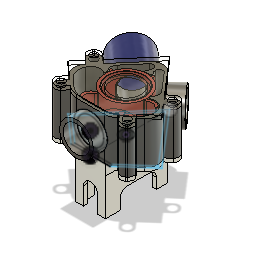
Air Transistor V4 (Autodesk Fusion 360 design; units mm, degrees)
Autodesk Fusion 360 part; units mm, degrees
sketch "Sketch1" plane through (0, 0, 0) normal (0, 1, 0) x (1, 0, 0)
  line L0 (-26.6187, 13.789) -> (0, 44.787)
  line L1 (-11, 0) -> (0, 0)
  line L2 (0, 44.787) -> (0, 0) construction
  line L3 (26.6187, 13.789) -> (0, 44.787)
  line L4 (11, 0) -> (0, 0)
  line L5 (-24.5168, 13.9343) -> (-10.4326, 1.5)
  line L6 (-26.6187, 13.789) -> (-11, 0)
  line L7 (-24.5168, 13.9343) -> (0, 42.4846)
  line L8 (-10.4326, 1.5) -> (0, 1.5)
  line L9 (24.5168, 13.9343) -> (10.4326, 1.5)
  line L10 (26.6187, 13.789) -> (11, 0)
  line L11 (10.4326, 1.5) -> (0, 1.5)
  line L12 (24.5168, 13.9343) -> (0, 42.4846)
  dimension "d70" = 1.5
  dimension "d71" = 1.5
  dimension "d72" = 22
  dimension "d73" = 1.5
  dimension "d85" = 0
  dimension "d86" = 0
  dimension "d87" = 0
  dimension "d88" = 0
  dimension "d121" = 0
  dimension "d122" = 0
  dimension "d123" = 0
  dimension "d124" = 0
  dimension "d131" = 0
  dimension "d132" = 0
  dimension "d133" = 0
  dimension "d134" = 0
  constraint coincident L1.end L2.end
  constraint horizontal L1
  constraint perpendicular L1 L2
  constraint symmetric L1.end L2 L4.end
  constraint symmetric L0.end L2 L3.end
  constraint parallel L5 L6
  constraint symmetric L2 L5.start L9.start
  constraint symmetric L2 L5.end L9.end
  constraint symmetric L2 L0.start L3.start
  constraint symmetric L2 L1.start L4.start
  constraint horizontal L8
  constraint horizontal L11
  constraint parallel L0 L7
  constraint parallel L3 L12
  measures "d70" distance of L5 L6
  measures "d71" distance of L0 L7
  measures "d72" distance of L1.start L4.start
  measures "d73" distance of L1 L8
extrude "Extrude1" add sketch "Sketch1" along normal blind 2 contours L5 L7 L8 L9 L11 L12 makes body 1
extrude "Extrude1'" add sketch "Sketch1" along normal blind 24 separate body makes body 2 in component "Casing"
ref_plane "WorkPlane1" through (0, 12, 0) normal (0, 0, 1) x (1, 0, 0)
sketch "Sketch2" plane through (0, 12, 0) normal (0, 0, 1) x (1, 0, 0)
  circle A0 centre (0, 0) radius 7.5
  circle A1 centre (0, 0) radius 9.5
  dimension "d9" = 15
  dimension "d10" = 2
  constraint coincident A0.centre A1.centre
  measures "d9" diameter of A0
  measures "d10" distance of A0 A1
extrude "Extrude3" add sketch "Sketch2" along normal blind 8 bodies 2 in component "Casing"
extrude "Extrude2" cut sketch "Sketch2" against normal blind 1.5 contours A0 bodies 2 in component "Casing"
ref_plane "WorkPlane2" through (13.3094, 12, -29.288) normal (0.758663, 0, -0.651483) x (-0.651483, 0, -0.758663)
sketch "Sketch3" plane through (13.3094, 12, -29.288) normal (0.758663, 0, -0.651483) x (-0.651483, 0, -0.758663)
  circle A0 centre (6.4293, 0) radius 7.5
  circle A1 centre (6.4293, 0) radius 9.5
  line L0 (0, 0) -> (60.3978, 0) construction
  line L1 (20.4293, -12) -> (20.4293, 12) construction
  dimension "d16" = 15
  dimension "d17" = 2
  dimension "d18" = 14
  constraint concentric A0 A1
  constraint coincident L0.start origin
  constraint horizontal L0
  constraint coincident A0.centre L0
  measures "d16" diameter of A0
  measures "d17" distance of A0 A1
  measures "d18" distance of A0.centre L1
extrude "Extrude4" add sketch "Sketch3" along normal blind 8 bodies 2 in component "Casing"
extrude "Extrude5" cut 1 faces at (7.7655, 9.2149, -35.7439) along direction (-0.758663, 0, 0.651483) blind 1.5 on bodies 2 bodies 2 in component "Casing"
ref_plane "WorkPlane3" through (-13.3094, 12, -29.288) normal (-0.758663, 0, -0.651483) x (-0.651483, 0, 0.758663)
sketch "Sketch4" plane through (-13.3094, 12, -29.288) normal (-0.758663, 0, -0.651483) x (-0.651483, 0, 0.758663)
  circle A0 centre (-6.4293, 0) radius 7.5
  circle A1 centre (-6.4293, 0) radius 9.5
  line L0 (0, 0) -> (-68.9221, 0) construction
  line L1 (-20.4293, -12) -> (-20.4293, 12) construction
  dimension "d24" = 15
  dimension "d25" = 2
  dimension "d26" = 14
  constraint concentric A0 A1
  constraint coincident L0.start origin
  constraint horizontal L0
  constraint coincident A0.centre L0
  measures "d24" diameter of A0
  measures "d25" distance of A0 A1
  measures "d26" distance of A0.centre L1
extrude "Extrude6" add sketch "Sketch4" along normal blind 8 bodies 2 in component "Casing"
extrude "Extrude7" cut 1 faces at (-8.723, 11.908, -34.6289) along direction (0.758663, 0, 0.651483) blind 1.5 on bodies 2 bodies 2 in component "Casing"
ref_plane "WorkPlane4" through (0, 2.5, -21.9923) normal (0, 1, 0) x (0, 0, 1)
sketch "Sketch5" plane through (0, 2.5, -33.891) normal (0, 1, 0) x (1, 0, 0)
  circle A0 centre (0, -13.7563) radius 12
  circle A1 centre (0, -13.7563) radius 10.5
  line L0 (0, 0) -> (0, -47.8942) construction
  dimension "d32" = 24
  dimension "d35" = 1.5
  constraint concentric A0 A1
  constraint coincident L0.start origin
  constraint vertical L0
  constraint coincident A0.centre L0
  measures "d32" diameter of A0
  measures "d35" distance of A0 A1
extrude "Extrude6'" add sketch "Sketch5" along normal blind 3 separate body contours A1 makes body 3
extrude "Extrude1''" add sketch "Sketch5" along normal up to surface (21.4 mm away) separate body makes body 4 in component "Exchanger"
ref_plane "WorkPlane6" through (0, 0, -21.9923) normal (0, 1, 0) x (1, 0, 0)
sketch "Sketch7" plane through (0, 0, -21.9857) normal (0, 1, 0) x (1, 0, 0)
  circle A0 centre (0, -1.8509) radius 3.5
  point P0 (0, -1.8509)
  dimension "d43" = 7
  constraint coincident P0 A0.centre
  measures "d43" diameter of A0
extrude "Extrude7'" cut sketch "Sketch7" along normal blind 2 bodies 1
copy_body "CutPasteBodies1" bodies 1 removing the originals makes body 5 in component "Casing"
copy_body "CutPasteBodies1'" bodies 3 removing the originals makes body 6 in component "Exchanger"
ref_plane "WorkPlane7" through (0, 5.5, -20.1347) normal (0, 1, 0) x (1, 0, 0)
sketch "Sketch8" plane through (0, 5.5, -20.1347) normal (0, 1, 0) x (1, 0, 0)
  circle A0 centre (0, 0) radius 3.5
  circle A1 centre (0, 0) radius 3.5
  constraint coincident A0.centre A1.centre
  constraint tangent A0 A1
extrude "Extrude2'" cut sketch "Sketch8" against normal blind 3 bodies 6 in component "Exchanger"
ref_plane "WorkPlane8" through (0, 21.1035, -30.6347) normal (0, 0, 1) x (-1, 0, 0)
sketch "Sketch9" plane through (0, 18.9317, -30.6347) normal (0, 0, 1) x (1, 0, 0)
  circle A0 centre (0, -5.7317) radius 8.5
  line L0 (0, 4.9683) -> (0, -16.4317) construction
  line L1 (-12, 4.9683) -> (12, 4.9683) construction
  line L2 (-8.5, -14.2317) -> (-6.5, -14.2317)
  line L3 (-6.5, -14.2317) -> (-6.5, 2.7683)
  line L4 (-6.5, 2.7683) -> (-8.5, 2.7683)
  line L5 (-8.5, 2.7683) -> (-8.5, -14.2317)
  line L6 (0, 2.7683) -> (-13.5085, 2.7683) construction
  line L7 (0, -14.2317) -> (-15.3531, -14.2317) construction
  line L8 (8.5, -14.2317) -> (6.5, -14.2317)
  line L9 (8.5, 2.7683) -> (8.5, -14.2317)
  line L10 (6.5, -14.2317) -> (6.5, 2.7683)
  line L11 (6.5, 2.7683) -> (8.5, 2.7683)
  point P0 (0, -16.4317)
  dimension "d56" = 17
  dimension "d232" = 2
  constraint coincident P0 L0.end
  constraint coincident L0.start L1
  constraint coincident L0 A0.centre
  constraint midpoint L0 A0.centre
  constraint coincident origin L0
  constraint horizontal L2
  constraint vertical L3
  constraint horizontal L4
  constraint vertical L5
  constraint tangent A0 L5
  constraint coincident L0 L6.start
  constraint coincident A0 L6.start
  constraint tangent A0 L6
  constraint coincident L0 L7.start
  constraint coincident A0 L7.start
  constraint tangent A0 L7
  constraint coincident L2.end L7
  constraint coincident L3.end L6
  constraint symmetric L0 L2.start L8.start
  constraint symmetric L0 L2.end L8.end
  constraint symmetric L0 L3.end L10.end
  constraint symmetric L0 L4.end L9.start
  measures "d56" diameter of A0
  measures "d232" distance of L3.end L4.end
extrude "Extrude3'" cut sketch "Sketch9" along normal mid plane 8 contours A0 L3 L10 bodies 4 in component "Exchanger"
ref_plane "WorkPlane10" through (0, 2, -21.9923) normal (0, 1, 0) x (0, 0, 1)
sketch "Sketch11" plane through (0, 2, -21.9857) normal (0, 1, 0) x (1, 0, 0)
  line L0 (-15.5611, 3.108) -> (-12.3, 0.1598)
  line L1 (-12.3, 0.1598) -> (-12.3, -1.8623)
  line L2 (-12.3, -1.8623) -> (-16.5628, 1.9915)
  line L3 (-16.5628, 1.9915) -> (-15.5611, 3.108)
  line L4 (0, 11.9053) -> (0, -35.9889)
  line L5 (12.3, 0.1598) -> (12.3, -1.8623)
  line L6 (15.5611, 3.108) -> (12.3, 0.1598)
  line L7 (12.3, -1.8623) -> (16.5628, 1.9915)
  line L8 (16.5628, 1.9915) -> (15.5611, 3.108)
  line L9 (-24.5168, -8.0514) -> (0, 20.4989)
  line L10 (-0.75, 19.6255) -> (-0.75, 11.9686)
  line L11 (-0.7497, 10.4669) -> (0, 10.5777)
  line L12 (0, 22.8013) -> (0, -21.9857)
  line L13 (0.75, 19.6255) -> (0.75, 11.9686)
  line L14 (0.7497, 10.4669) -> (0, 10.5777)
  line L15 (-0.75, 19.6255) -> (0, 20.4989)
  line L16 (0, 20.4989) -> (0.75, 19.6255)
  circle A0 centre (0, -1.8509) radius 12 construction
  line L17 (-0.7497, 10.4669) -> (-1.9495, 10.2897)
  line L18 (-1.9495, 10.2897) -> (-1.9495, 11.7897)
  line L19 (-1.9495, 11.7897) -> (-0.75, 11.9686)
  line L20 (1.9495, 11.7897) -> (0.75, 11.9686)
  line L21 (1.9495, 10.2897) -> (1.9495, 11.7897)
  line L22 (0.7497, 10.4669) -> (1.9495, 10.2897)
  line L23 (-12.3, -1.8623) -> (-12, -1.8623) construction
  line L24 (-1.9495, 10.2897) -> (-1.9495, 9.9897) construction
  dimension "d67" = 1.5
  dimension "d100" = 1.5
  dimension "d125" = 1.5
  dimension "d198" = 0.3
  dimension "d199" = 0.3
  constraint vertical L1
  constraint parallel L0 L2
  constraint symmetric L0.start L4 L6.start
  constraint symmetric L0.end L4 L5.start
  constraint symmetric L1.end L4 L5.end
  constraint symmetric L2.end L4 L7.end
  constraint coincident L9 L10.start
  constraint vertical L10
  constraint coincident L4 L11.end
  constraint symmetric L10.start L12 L13.start
  constraint symmetric L11.start L12 L14.start
  constraint coincident L9.end L15.end
  constraint parallel L11 L17
  constraint parallel L10 L18
  constraint equal L17 L19
  constraint symmetric L12 L17.end L21.start
  constraint symmetric L12 L18.end L20.start
  constraint symmetric L12 L10.end L13.end
  constraint coincident A0 L23.end
  constraint perpendicular L1 L23
  constraint coincident A0 L24.end
  constraint parallel L18 L24
  measures "d67" distance of L0 L2
  measures "d100" distance of L10 L13
  measures "d125" distance of L17.end L18.end
  measures "d198" distance of L1.end L23.end
  measures "d199" distance of L17.end L24.end
extrude "Extrude8" add sketch "Sketch11" along normal up to surface (22 mm away) bodies 2 5 in component "Casing"
fillet "Fillet1" radius 8 2 edges at (-24.5168, 13, -13.9343) (24.5168, 13, -13.9343) on bodies 2 in component "Casing"
fillet "Fillet2" radius 14.5 2 edges at (-10.4326, 13, -1.5) (10.4326, 13, -1.5) on bodies 2 in component "Casing"
fillet "Fillet3" radius 2 2 edges at (-0.75, 13, -41.6112) (0.75, 13, -41.6112) on bodies 2 in component "Casing"
fillet "Fillet4" radius 5.5 2 edges at (16.1856, 13, -23.6362) (-16.1856, 13, -23.6362) on bodies 2 in component "Casing"
fillet "Fillet5" radius 4 2 edges at (-15.208, 13, -24.7745) (15.208, 13, -24.7745) on bodies 2 in component "Casing"
ref_plane "WorkPlane11" through (0, 13.4776, -9.6347) normal (0, 0, -1) x (1, 0, 0)
sketch "Sketch12" plane through (0, 12.0321, -9.6347) normal (0, 0, -1) x (1, 0, 0)
  circle A0 centre (0, -1.1679) radius 7.5
  line L0 (0, 9.5321) -> (0, -11.8679) construction
  line L1 (12, -11.8679) -> (-12, -11.8679) construction
  point P0 (0, 9.5321)
  dimension "d94" = 15
  constraint vertical L0
  constraint coincident L0.end L1
  constraint coincident P0 L0.start
  constraint coincident A0.centre L0
  constraint midpoint A0.centre L0
  measures "d94" diameter of A0
extrude "Extrude5'" cut sketch "Sketch12" along normal mid plane 8 bodies 4 in component "Exchanger"
fillet "Fillet1'" radius 2 1 edges at (-9.7894, 5.5, -16.3378) on bodies 6 in component "Exchanger"
ref_plane "WorkPlane13" through (0, 5.5, -20.1347) normal (0, 1, 0) x (1, 0, 0)
sketch "Sketch14" plane through (0, 5.5, -20.1347) normal (0, 1, 0) x (1, 0, 0)
  circle A0 centre (0, 0) radius 3.7
  circle A1 centre (0, 0) radius 3.5
  line L0 (3.7, 8.5) -> (-3.7, 8.5)
  line L1 (-3.7, 8.5) -> (-3.7, -8.5)
  line L2 (-3.7, -8.5) -> (3.7, -8.5)
  line L3 (3.7, -8.5) -> (3.7, 8.5)
  line L4 (3.7, 8.5) -> (-3.7, -8.5) construction
  line L5 (-3.7, 8.5) -> (3.7, -8.5) construction
  circle A2 centre (0, 0) radius 8.5
  line L6 (-3.7, 8.5) -> (-2.5, 8.5)
  line L7 (-2.5, 8.5) -> (-2.5, 4.5)
  line L8 (-2.5, 4.5) -> (-3.7, 4.5)
  line L9 (-3.7, 4.5) -> (-3.7, 8.5)
  line L10 (0, 24.6522) -> (0, -20.1347)
  line L11 (3.7, 8.5) -> (2.5, 8.5)
  line L12 (2.5, 4.5) -> (3.7, 4.5)
  line L13 (3.7, 4.5) -> (3.7, 8.5)
  line L14 (2.5, 8.5) -> (2.5, 4.5)
  line L15 (0, 0) -> (-15.4178, 0) construction
  line L16 (-2.5, -8.5) -> (-2.5, -4.5)
  line L17 (-3.7, -8.5) -> (-2.5, -8.5)
  line L18 (3.7, -8.5) -> (-3.7, -8.5)
  line L19 (2.5, -8.5) -> (2.5, -4.5)
  line L20 (-3.7, -4.5) -> (-3.7, -8.5)
  line L21 (-2.5, -4.5) -> (-3.7, -4.5)
  line L22 (3.7, -4.5) -> (3.7, -8.5)
  line L23 (2.5, -4.5) -> (3.7, -4.5)
  line L24 (3.7, -8.5) -> (2.5, -8.5)
  dimension "d108" = 0.2
  dimension "d256" = 5
  dimension "d257" = 4
  constraint coincident A0.centre A1.centre
  constraint horizontal L0
  constraint perpendicular L0 L1
  constraint parallel L0 L2
  constraint parallel L1 L3
  constraint coincident L4 A0.centre
  constraint coincident L5 A0.centre
  constraint tangent A0 L1
  constraint tangent L0 A2
  constraint horizontal L6
  constraint vertical L7
  constraint horizontal L8
  constraint vertical L9
  constraint symmetric L0.end L10 L0.start
  constraint symmetric L6.end L10 L11.end
  constraint symmetric L7.end L10 L12.start
  constraint symmetric L8.end L10 L12.end
  constraint perpendicular L10 L15
  constraint symmetric L0.start L15 L2.end
  constraint symmetric L0.end L15 L1.end
  constraint symmetric L6.end L15 L16.start
  constraint symmetric L7.end L15 L16.end
  constraint symmetric L8.end L15 L20.start
  constraint symmetric L12.start L15 L19.end
  constraint symmetric L12.end L15 L22.start
  constraint symmetric L11.end L15 L19.start
  measures "d108" distance of A0 A1
  measures "d256" distance of L6.end L11.end
  measures "d257" distance of L12.start L11.end
extrude "Extrude6''" cut sketch "Sketch14" against normal blind 1 contours A0 A1 L10 | A0 L3 A2 L10 L19 L23 | A0 L3 A2 L10 L12 L14 | A0 A1 L10 | A0 L1 A2 L7 L8 L10 | A0 L1 A2 L10 L16 L21 bodies 6 in component "Exchanger"
fillet "Fillet8" radius 0.75 2 edges at (1.9495, 13, -33.7753) (-1.9495, 13, -33.7753) on bodies 2 in component "Casing"
fillet "Fillet9" radius 6.5 1 edges at (0, 13, -32.5634) on bodies 2 in component "Casing"
fillet "Fillet10" radius 3.5 2 edges at (0.75, 13, -33.9543) (-0.75, 13, -33.9543) on bodies 2 in component "Casing"
ref_plane "WorkPlane14" through (0, 0, -21.9923) normal (0, 1, 0) x (1, 0, 0)
sketch "Sketch15" plane through (0, 0, -21.9923) normal (0, 1, 0) x (1, 0, 0)
  circle A0 centre (0, -1.8575) radius 8.5
  point P0 (0, -1.8575)
  dimension "d136" = 17
  constraint coincident P0 A0.centre
  measures "d136" diameter of A0
extrude "Extrude10" cut sketch "Sketch15" along normal up to surface (2 mm away) bodies 2 in component "Casing"
ref_plane "WorkPlane15" through (0, 24, -22.3935) normal (0, 1, 0) x (0, 0, 1)
sketch "Sketch16" plane through (0, 24, -20.5211) normal (0, 1, 0) x (1, 0, 0)
  line L0 (0, 24.2659) -> (-26.6187, -6.7321)
  line L1 (-26.6187, -6.7321) -> (-11, -20.5211)
  line L2 (-11, -20.5211) -> (11, -20.5211)
  line L3 (11, -20.5211) -> (26.6187, -6.7321)
  line L4 (26.6187, -6.7321) -> (0, 24.2659)
  point P0 (0, 24.2659)
  point P1 (-26.6187, -6.7321)
  point P2 (11, -20.5211)
  point P3 (26.6187, -6.7321)
  point P4 (-11, -20.5211)
  constraint horizontal L2
  constraint coincident P0 L0.start
  constraint coincident P1 L0.end
  constraint coincident P2 L2.end
  constraint coincident P3 L3.end
  constraint coincident P4 L1.end
ref_plane "WorkPlane16" through (0, 24, -22.3935) normal (0, 1, 0) x (0, 0, 1)
sketch "Sketch17" plane through (0, 24, -20.5211) normal (0, 1, 0) x (1, 0, 0)
  line L0 (-21.9096, -1.2482) -> (-27.2202, 3.3122)
  line L1 (-27.2202, 3.3122) -> (-22.6598, 8.6228)
  line L2 (-22.6598, 8.6228) -> (-17.3492, 4.0624)
  line L3 (-26.6187, -6.7321) -> (0, 24.2659)
  line L4 (0, 24.2659) -> (0, -20.5211)
  line L5 (27.2202, 3.3122) -> (22.6598, 8.6228)
  line L6 (22.6598, 8.6228) -> (17.3492, 4.0624)
  line L7 (21.9096, -1.2482) -> (27.2202, 3.3122)
  line L8 (17.3492, 4.0624) -> (21.9096, -1.2482)
  circle A0 centre (-22.2847, 3.6873) radius 2.1
  line L9 (-27.2202, 3.3122) -> (-17.3492, 4.0624) construction
  line L10 (-22.6598, 8.6228) -> (-21.9096, -1.2482) construction
  circle A1 centre (22.2847, 3.6873) radius 2.1
  line L11 (-18.9871, -13.4697) -> (-23.6199, -18.7173)
  line L12 (-23.6199, -18.7173) -> (-18.3723, -23.3501)
  line L13 (-18.3723, -23.3501) -> (-13.7395, -18.1026)
  line L14 (-13.7395, -18.1026) -> (-18.9871, -13.4697)
  line L15 (-26.6187, -6.7321) -> (-11, -20.5211)
  line L16 (-23.6199, -18.7173) -> (-22.9202, -19.3351) construction
  line L17 (-13.7395, -18.1026) -> (-23.6199, -18.7173) construction
  line L18 (-18.9871, -13.4697) -> (-18.3723, -23.3501) construction
  circle A2 centre (-18.6797, -18.4099) radius 2.1
  line L19 (18.3723, -23.3501) -> (13.7395, -18.1026)
  line L20 (13.7395, -18.1026) -> (18.9871, -13.4697)
  line L21 (13.7395, -18.1026) -> (23.6199, -18.7173) construction
  line L22 (18.9871, -13.4697) -> (18.3723, -23.3501) construction
  line L23 (18.9871, -13.4697) -> (23.6199, -18.7173)
  line L24 (23.6199, -18.7173) -> (22.9202, -19.3351) construction
  line L25 (23.6199, -18.7173) -> (18.3723, -23.3501)
  circle A3 centre (18.6797, -18.4099) radius 2.1
  point P0 (-22.2847, 3.6873)
  point P1 (-18.6797, -18.4099)
  point P2 (18.6797, -18.4099)
  point P3 (11, -20.5211)
  dimension "d149" = 4.2
  dimension "d150" = 7
  dimension "d151" = 7
  constraint perpendicular L0 L1
  constraint perpendicular L1 L2
  constraint coincident L0.start L3
  constraint coincident L2.end L3
  constraint parallel L1 L3
  constraint symmetric L0.start L4 L7.start
  constraint symmetric L0.end L4 L5.start
  constraint symmetric L1.end L4 L5.end
  constraint symmetric L2.end L4 L6.end
  constraint perpendicular L7 L8
  constraint midpoint L9 P0
  constraint coincident P0 A0.centre
  constraint symmetric L4 A0 A1
  constraint perpendicular L12 L13
  constraint perpendicular L11 L14
  constraint perpendicular L13 L14
  constraint coincident L13.end L15
  constraint coincident L11.start L15
  constraint equal L0 L11
  constraint equal L1 L12
  constraint coincident L12 L16.end
  constraint midpoint L18 P1
  constraint coincident P1 A2.centre
  constraint equal A0 A2
  constraint symmetric L4 L11.start L20.end
  constraint symmetric L4 L11.end L21.end
  constraint symmetric L4 L12.end L19.start
  constraint symmetric L4 L13.end L19.end
  constraint symmetric L4 L15.end P3
  constraint symmetric L4 L16.end L24.end
  constraint symmetric L4 P1 P2
  constraint symmetric L4 A2 A3
  measures "d149" diameter of A0
  measures "d150" distance of L0.end L1.end
  measures "d151" distance of L0.start L0.end
extrude "Extrude11" add sketch "Sketch17" against normal blind 24 bodies 2 in component "Casing"
ref_plane "WorkPlane18" through (0, 24, -20.979) normal (0, 1, 0) x (0, 0, 1)
sketch "Sketch19" plane through (0, 24, -19.1066) normal (0, 1, 0) x (1, 0, 0)
  line L0 (-26.6187, -5.3176) -> (-18.9871, -12.0552)
  line L1 (-18.9871, -12.0552) -> (-23.5757, -17.3988)
  line L2 (-23.5757, -17.3988) -> (-18.3379, -21.8966)
  line L3 (-18.3379, -21.8966) -> (-13.7395, -16.6881)
  line L4 (-11, -19.1066) -> (-2.9302, -19.1066)
  line L5 (-2.9302, -19.1066) -> (0, -19.1066)
  line L6 (0, -19.1066) -> (0, 25.6803)
  line L7 (-17.3492, 5.4769) -> (-22.6598, 10.0373)
  line L8 (-22.6598, 10.0373) -> (-27.2202, 4.7267)
  line L9 (-27.2202, 4.7267) -> (-21.9096, 0.1663)
  line L10 (0, 25.6803) -> (-17.3492, 5.4769)
  line L11 (-21.9096, 0.1663) -> (-26.6187, -5.3176)
  line L12 (-13.7395, -16.6881) -> (-11, -19.1066)
  line L13 (-18.3723, -21.9356) -> (-13.7395, -16.6881)
  line L14 (-26.6187, -5.3176) -> (-11, -19.1066)
  line L15 (-18.9871, -12.0552) -> (-23.6199, -17.3028)
  line L16 (-23.6199, -17.3028) -> (-18.3723, -21.9356) construction
  line L17 (-26.6187, -5.3176) -> (0, 25.6803) construction
  line L18 (-21.9096, 0.1663) -> (-27.2202, 4.7267) construction
  line L19 (-22.6598, 10.0373) -> (-17.3492, 5.4769) construction
  line L20 (-27.2202, 4.7267) -> (-22.6598, 10.0373) construction
  line L21 (0, 25.6803) -> (0, 31.3703) construction
  line L22 (11, -19.1066) -> (2.9302, -19.1066)
  line L23 (13.7395, -16.6881) -> (11, -19.1066)
  line L24 (21.9096, 0.1663) -> (27.2202, 4.7267) construction
  line L25 (0, 25.6803) -> (17.3492, 5.4769)
  line L26 (26.6187, -5.3176) -> (11, -19.1066)
  line L27 (26.6187, -5.3176) -> (18.9871, -12.0552)
  line L28 (0, -19.1066) -> (0, 25.6803)
  line L29 (18.9871, -12.0552) -> (23.5757, -17.3988)
  line L30 (22.6598, 10.0373) -> (17.3492, 5.4769) construction
  line L31 (18.9871, -12.0552) -> (23.6199, -17.3028)
  line L32 (27.2202, 4.7267) -> (21.9096, 0.1663)
  line L33 (23.5757, -17.3988) -> (18.3379, -21.8966)
  line L34 (18.3723, -21.9356) -> (13.7395, -16.6881)
  line L35 (26.6187, -5.3176) -> (0, 25.6803) construction
  line L36 (21.9096, 0.1663) -> (26.6187, -5.3176)
  line L37 (2.9302, -19.1066) -> (0, -19.1066)
  line L38 (18.3379, -21.8966) -> (13.7395, -16.6881)
  line L39 (17.3492, 5.4769) -> (22.6598, 10.0373)
  line L40 (27.2202, 4.7267) -> (22.6598, 10.0373) construction
  line L41 (22.6598, 10.0373) -> (27.2202, 4.7267)
  line L42 (23.6199, -17.3028) -> (18.3723, -21.9356) construction
  circle A0 centre (-22.2847, 5.1018) radius 2.1
  circle A1 centre (-18.6797, -16.9954) radius 2.1
  circle A2 centre (18.6797, -16.9954) radius 2.1
  circle A3 centre (22.2847, 5.1018) radius 2.1
  circle A4 centre (-22.2847, 5.1018) radius 2.1
  circle A5 centre (-18.6797, -16.9954) radius 2.1
  circle A6 centre (18.6797, -16.9954) radius 2.1
  circle A7 centre (22.2847, 5.1018) radius 2.1
  point P0 (0, 25.6803)
  point P1 (0, -19.1066)
  point P2 (-21.2129, -19.4278)
  point P3 (-24.8897, 7.4406)
  point P4 (0, 25.6803)
  point P5 (24.8897, 7.4406)
  point P6 (21.2129, -19.4278)
  point P7 (0, 25.6803)
  point P8 (0, -19.1066)
  constraint parallel L1 L10
  constraint perpendicular L1 L2
  constraint horizontal L5
  constraint perpendicular L7 L10
  constraint perpendicular L7 L8
  constraint perpendicular L9 L10
  constraint collinear L10 L11
  constraint coincident P7 P4
  constraint coincident P8 P1
  constraint coincident L3.end L12.start
  constraint coincident L3.end L13
  constraint coincident L3.end L14
  constraint coincident L4.start L12.end
  constraint coincident L3 L13.start
  constraint coincident L0.end L15
  constraint coincident L0.end L14
  constraint coincident P2 L16
  constraint coincident L2 P2
  constraint coincident L7.start L17
  constraint coincident L9.end L18
  constraint coincident L7.start L19
  constraint coincident P3 L20
  constraint coincident L8 P3
  constraint coincident L0.start L11.end
  constraint parallel L6 L21
  constraint symmetric P7 L21 P4
  constraint symmetric L0.start L21 L26.start
  constraint symmetric L0.end L21 L27.end
  constraint symmetric L1.end L21 L29.end
  constraint symmetric L2.end L21 L33.end
  constraint symmetric L4.end L21 L22.end
  constraint symmetric P8 L21 P1
  constraint symmetric L7.start L21 L25.end
  constraint symmetric L7.end L21 L30.start
  constraint symmetric L8.end L21 L24.end
  constraint symmetric L9.end L21 L24.start
  constraint symmetric L3.end L21 L23.start
  constraint symmetric L4.start L21 L22.start
  constraint symmetric L13.start L21 L34.start
  constraint symmetric L15.end L21 L31.end
  constraint symmetric P2 L21 P6
  constraint symmetric P3 L21 P5
  constraint tangent A0 A4
  constraint tangent A1 A5
  constraint tangent A2 A6
  constraint tangent A3 A7
  constraint equal A0 A4
  constraint equal A1 A5
  constraint equal A2 A6
  constraint equal A3 A7
extrude "Extrude1'''" add sketch "Sketch19" along normal blind 2 separate body makes body 7 in component "Roof"
ref_plane "WorkPlane19" through (0, 0, -20.979) normal (0, -1, 0) x (-1, 0, 0)
sketch "Sketch20" plane through (0, 0, -19.1066) normal (0, -1, 0) x (1, 0, 0)
  line L0 (-23.6199, 17.3028) -> (-18.3723, 21.9356)
  line L1 (-18.3723, 21.9356) -> (-13.7395, 16.6881)
  line L2 (-13.7395, 16.6881) -> (-11, 19.1066)
  line L3 (-11, 19.1066) -> (0, 19.1066)
  line L4 (-23.6199, 17.3028) -> (-18.9871, 12.0552)
  line L5 (-18.9871, 12.0552) -> (-26.6187, 5.3176)
  line L6 (-26.6187, 5.3176) -> (-21.9096, -0.1663)
  line L7 (-21.9096, -0.1663) -> (-27.2202, -4.7267)
  line L8 (-27.2202, -4.7267) -> (-22.6598, -10.0373)
  line L9 (-22.6598, -10.0373) -> (-17.3492, -5.4769)
  line L10 (-17.3492, -5.4769) -> (0, -25.6803)
  line L11 (0, -25.6803) -> (0, 19.1066)
  line L12 (-11, 19.1066) -> (0, 19.1066)
  line L13 (-13.7395, 16.6881) -> (-18.3723, 21.9356)
  line L14 (-26.6187, 5.3176) -> (-11, 19.1066)
  line L15 (-18.3723, 21.9356) -> (-23.6199, 17.3028)
  line L16 (-23.6199, 17.3028) -> (-18.9871, 12.0552)
  line L17 (-21.9096, -0.1663) -> (-27.2202, -4.7267)
  line L18 (-26.6187, 5.3176) -> (0, -25.6803)
  line L19 (-27.2202, -4.7267) -> (-22.6598, -10.0373)
  line L20 (-22.6598, -10.0373) -> (-17.3492, -5.4769)
  line L21 (0, -14.7844) -> (0, 33.1099)
  line L22 (21.9096, -0.1663) -> (27.2202, -4.7267)
  line L23 (26.6187, 5.3176) -> (11, 19.1066)
  line L24 (22.6598, -10.0373) -> (17.3492, -5.4769)
  line L25 (0, -25.6803) -> (0, 19.1066)
  line L26 (17.3492, -5.4769) -> (0, -25.6803)
  line L27 (26.6187, 5.3176) -> (0, -25.6803)
  line L28 (27.2202, -4.7267) -> (22.6598, -10.0373)
  line L29 (18.9871, 12.0552) -> (26.6187, 5.3176)
  line L30 (21.9096, -0.1663) -> (27.2202, -4.7267)
  line L31 (22.6598, -10.0373) -> (17.3492, -5.4769)
  line L32 (27.2202, -4.7267) -> (22.6598, -10.0373)
  line L33 (26.6187, 5.3176) -> (21.9096, -0.1663)
  line L34 (13.7395, 16.6881) -> (18.3723, 21.9356)
  line L35 (23.6199, 17.3028) -> (18.9871, 12.0552)
  line L36 (18.3723, 21.9356) -> (23.6199, 17.3028)
  line L37 (11, 19.1066) -> (0, 19.1066)
  line L38 (11, 19.1066) -> (0, 19.1066)
  line L39 (18.3723, 21.9356) -> (13.7395, 16.6881)
  line L40 (23.6199, 17.3028) -> (18.3723, 21.9356)
  line L41 (23.6199, 17.3028) -> (18.9871, 12.0552)
  line L42 (13.7395, 16.6881) -> (11, 19.1066)
  circle A0 centre (-18.6797, 16.9954) radius 2.1
  circle A1 centre (-22.2847, -5.1018) radius 2.1
  circle A2 centre (18.6797, 16.9954) radius 2.1
  circle A3 centre (22.2847, -5.1018) radius 2.1
  circle A4 centre (-18.6797, 16.9954) radius 2.1
  circle A5 centre (18.6797, 16.9954) radius 2.1
  circle A6 centre (-22.2847, -5.1018) radius 2.1
  circle A7 centre (22.2847, -5.1018) radius 2.1
  circle A8 centre (0, -1.0281) radius 8.5
  circle A9 centre (0, -1.0281) radius 8.5
  point P0 (0, -1.0281)
  point P1 (0, -1.0281)
  constraint horizontal L3
  constraint parallel L6 L10
  constraint vertical L11
  constraint coincident L11 P1
  constraint coincident L3.end L12
  constraint coincident L2.end L3.start
  constraint coincident L1.end L13
  constraint coincident L1.end L14
  constraint coincident L0.end L13
  constraint coincident L0.end L15
  constraint perpendicular L0 L1
  constraint perpendicular L0 L4
  constraint perpendicular L4 L5
  constraint coincident L4.end L16
  constraint coincident L5.end L6.start
  constraint coincident L6.end L17
  constraint coincident L6.end L18
  constraint perpendicular L7 L18
  constraint perpendicular L8 L9
  constraint perpendicular L7 L8
  constraint coincident L7.end L19
  constraint coincident L8.end L20
  constraint coincident L9.end L10.start
  constraint symmetric L0.start L21 L35.start
  constraint symmetric L0.end L21 L34.end
  constraint symmetric L1.end L21 L34.start
  constraint symmetric L2.end L21 L23.end
  constraint symmetric L3.end L21 L11.end
  constraint symmetric L4.end L21 L29.start
  constraint symmetric L5.end L21 L23.start
  constraint symmetric L6.end L21 L22.start
  constraint symmetric L7.end L21 L22.end
  constraint symmetric L8.end L21 L24.start
  constraint symmetric L9.end L21 L24.end
  constraint symmetric L10.end L21 L11.start
  constraint symmetric P1 L21 P0
  constraint tangent A0 A4
  constraint tangent A2 A5
  constraint tangent A1 A6
  constraint tangent A3 A7
  constraint equal A0 A4
  constraint equal A2 A5
  constraint equal A3 A7
  constraint equal A1 A6
  constraint coincident P1 P0
  constraint tangent A8 A9
extrude "Extrude1''''" add sketch "Sketch20" sketch "Sketch1" along normal blind 2 separate body contours L0 L1 L4 L13 L14 L15 L16 | L2 L3 L5 L6 L10 L11 L12 L14 L18 L21 L25 A8 A9 | L7 L8 L9 L17 L18 L19 L20 | L11 L21 L23 L25 L26 L27 L29 L33 L37 L38 L42 A8 A9 | L23 L34 L35 L36 L39 L40 L41 | L22 L24 L27 L28 L30 L31 L32 of sketch 2 makes body 8 in component "Motor Casing"
fillet "Fillet1''" radius 8 2 edges at (-11, -1, 0) (11, -1, 0) on bodies 8 in component "Motor Casing"
fillet "Fillet17" radius 8 2 edges at (-11, 12, 0) (11, 12, 0) on bodies 2 in component "Casing"
fillet "Fillet4'" radius 8 2 edges at (-11, 25, 0) (11, 25, 0) on bodies 7 in component "Roof"
fillet "Fillet3'" radius 3 8 edges at (-27.2202, -1, -23.8333) (-22.6598, -1, -29.144) (-23.6199, -1, -1.8038) (-18.3723, -1, 2.829) (23.6199, -1, -1.8038) (18.3723, -1, 2.829) (22.6598, -1, -29.144) (27.2202, -1, -23.8333) on bodies 8 in component "Motor Casing"
fillet "Fillet19" radius 3 8 edges at (-27.2202, 12, -23.8333) (-22.6598, 12, -29.144) (-23.6199, 12, -1.8038) (-18.3723, 12, 2.829) (23.6199, 12, -1.8038) (18.3723, 12, 2.829) (27.2202, 12, -23.8333) (22.6598, 12, -29.144) on bodies 2 in component "Casing"
fillet "Fillet6" radius 3 8 edges at (-27.2202, 25, -23.8333) (-22.6598, 25, -29.144) (-23.5757, 25, -1.7078) (-18.3379, 25, 2.79) (23.5757, 25, -1.7078) (18.3379, 25, 2.79) (22.6598, 25, -29.144) (27.2202, 25, -23.8333) on bodies 7 in component "Roof"
ref_plane "WorkPlane20" through (0, -2, -20.979) normal (0, -1, 0) x (1, 0, 0)
sketch "Sketch21" plane through (0, -2, -19.1066) normal (0, -1, 0) x (1, 0, 0)
  line L0 (-8.5, 19.1066) -> (-6.25, 19.1066)
  line L1 (-6.25, 19.1066) -> (-6.25, -18.4021)
  line L2 (-6.25, -18.4021) -> (-8.5, -15.782)
  line L3 (-8.5, -15.782) -> (-8.5, 19.1066)
  line L4 (0, -25.6803) -> (0, 19.1066)
  line L5 (-11, 19.1066) -> (0, 19.1066)
  line L6 (-26.6187, 5.3176) -> (0, -25.6803)
  line L7 (8.5, -15.782) -> (8.5, 19.1066)
  line L8 (6.25, 19.1066) -> (6.25, -18.4021)
  line L9 (8.5, 19.1066) -> (6.25, 19.1066)
  line L10 (6.25, -18.4021) -> (8.5, -15.782)
  circle A0 centre (0, -1.0281) radius 8.5
  line L11 (-6.25, 19.1066) -> (6.25, 19.1066)
  line L12 (6.25, 19.1066) -> (6.25, 16.8566)
  line L13 (6.25, 16.8566) -> (-6.25, 16.8566)
  line L14 (-6.25, 16.8566) -> (-6.25, 19.1066)
  point P0 (11, 19.1066)
  dimension "d180" = 6.25
  constraint horizontal L0
  constraint vertical L1
  constraint vertical L3
  constraint coincident L0.end L5
  constraint coincident L2.end L6
  constraint symmetric L0.start L4 L7.end
  constraint symmetric L0.end L4 L8.start
  constraint symmetric L1.end L4 L8.end
  constraint symmetric L2.end L4 L7.start
  constraint symmetric L4 L5.start P0
  constraint coincident L1.end L6
  constraint tangent L3 A0
  constraint horizontal L11
  constraint vertical L12
  constraint horizontal L13
  constraint vertical L14
  constraint equal L0 L14
  constraint coincident L0.end L1.start
  constraint coincident L8.start L9.end
  measures "d180" distance of L1 L4
extrude "Extrude2''" add sketch "Sketch21" along normal blind 25 and the other way up to surface (2 mm away) contours L0 L1 L3 L5 A0 L14 | L1 L4 L5 L11 L13 L14 | L1 L2 L3 L6 A0 | L1 A0 | L4 L8 L11 L12 L13 | L7 L8 L9 A0 L12 | L8 A0 | L7 L8 L10 A0 bodies 8 in component "Motor Casing"
chamfer "Chamfer1" distance 4 angle 45 2 edges at (-8.5, -2, -17.453) (8.5, -2, -17.453) on bodies 8 in component "Motor Casing"
ref_plane "WorkPlane21" through (0, -27, -18.7544) normal (0, -1, 0) x (0, 0, -1)
sketch "Sketch22" plane through (0, -27, -18.7544) normal (0, -1, 0) x (1, 0, 0)
  line L0 (-4, 18.7544) -> (4, 18.7544)
  line L1 (4, 18.7544) -> (4, 16.5044)
  line L2 (4, 16.5044) -> (-4, 16.5044)
  line L3 (-4, 16.5044) -> (-4, 18.7544)
  line L4 (-6.25, 16.5044) -> (6.25, 16.5044)
  line L5 (11, 18.7544) -> (0, 18.7544)
  line L6 (0, 18.7544) -> (0, 12.1795) construction
  point P0 (0, 18.7544)
  dimension "d188" = 8
  constraint horizontal L0
  constraint vertical L1
  constraint horizontal L2
  constraint vertical L3
  constraint coincident L2.end L4
  constraint coincident L0.end L5
  constraint midpoint L0 P0
  constraint perpendicular L0 L6
  constraint coincident L6 P0
  measures "d188" distance of L0.start L0.end
extrude "Extrude3''" cut sketch "Sketch22" against normal blind 14 bodies 8 in component "Motor Casing"
fillet "Fillet4''" radius 4 2 edges at (4, -13, -1.125) (-4, -13, -1.125) on bodies 8 in component "Motor Casing"
ref_plane "WorkPlane22" through (0, -27, -18.7544) normal (0, -1, 0) x (0, 0, -1)
sketch "Sketch23" plane through (-6.25, -27, -18.7544) normal (0, -1, 0) x (1, 0, 0)
  line L0 (-2.25, 10.5044) -> (0, 10.5044)
  line L1 (0, 10.5044) -> (0, -10.1342)
  line L2 (0, -10.1342) -> (-2.25, -10.1342)
  line L3 (-2.25, -10.1342) -> (-2.25, 10.5044)
  line L4 (-2.25, 18.7544) -> (-2.25, -16.1342)
  line L5 (0, -18.7544) -> (0, 16.5044)
  line L6 (6.25, -26.0326) -> (6.25, 18.7544)
  line L7 (12.5, -10.1342) -> (14.75, -10.1342)
  line L8 (14.75, 10.5044) -> (12.5, 10.5044)
  line L9 (12.5, 10.5044) -> (12.5, -10.1342)
  line L10 (14.75, -10.1342) -> (14.75, 10.5044)
  point P0 (12.5, 0)
  dimension "d193" = 6
  dimension "d194" = 6
  constraint horizontal L0
  constraint vertical L1
  constraint horizontal L2
  constraint vertical L3
  constraint coincident L0.start L4
  constraint coincident L0.end L5
  constraint symmetric origin L6 P0
  constraint symmetric L0.start L6 L8.start
  constraint symmetric L0.end L6 L8.end
  constraint symmetric L1.end L6 L7.start
  constraint symmetric L2.end L6 L7.end
  measures "d193" distance of L0.end L5.end
  measures "d194" distance of L2.end L4.end
extrude "Extrude4'" cut sketch "Sketch23" against normal blind 10 bodies 8 in component "Motor Casing"
fillet "Fillet5'" radius 4 4 edges at (7.375, -17, -8.25) (7.375, -17, -28.8886) (-7.375, -17, -8.25) (-7.375, -17, -28.8886) on bodies 8 in component "Motor Casing"
ref_plane "WorkPlane24" through (-15.1901, 12, -39.3776) normal (-0.758663, 0, -0.651483) x (-0.651483, 0, 0.758663)
sketch "Sketch25" plane through (-15.1901, 12, -39.3776) normal (-0.758663, 0, -0.651483) x (-0.651483, 0, 0.758663)
  circle A0 centre (0, 0) radius 9.6
  circle A1 centre (0, 0) radius 11.1
  circle A2 centre (0, 0) radius 9.5
  dimension "d205" = 1.5
  dimension "d206" = 0.1
  constraint coincident A0.centre A1.centre
  measures "d205" distance of A0 A1
  measures "d206" distance of A0 A2
extrude "Extrude1'''''" add sketch "Sketch25" along normal blind -7.9 and the other way blind -14 separate body contours A1 makes body 9 in component "Adapter 15-15"
ref_plane "WorkPlane25" through (0, -2, -20.979) normal (0, -1, 0) x (1, 0, 0)
sketch "Sketch26" plane through (0, -2, -8.3119) normal (0, -1, 0) x (1, 0, 0)
  line L0 (-6.25, 6.0619) -> (6.25, 6.0619)
  line L1 (6.25, 6.0619) -> (6.25, 3.0619)
  line L2 (6.25, 3.0619) -> (-6.25, 3.0619)
  line L3 (-6.25, 3.0619) -> (-6.25, 6.0619)
  point P0 (-6.25, 6.0619)
  point P1 (6.25, 6.0619)
  dimension "d211" = 3
  constraint horizontal L0
  constraint vertical L1
  constraint horizontal L2
  constraint vertical L3
  constraint coincident P0 L0.start
  constraint coincident P1 L0.end
  measures "d211" distance of P1 L1.end
extrude "Extrude5''" add sketch "Sketch26" along normal blind 7 bodies 8 in component "Motor Casing"
chamfer "Chamfer2" distance 3 angle 45 1 edges at (0, -9, -2.25) on bodies 8 in component "Motor Casing"
ref_plane "WorkPlane26" through (0, 23.9, -20.1347) normal (0, 1, 0) x (0, 0, 1)
sketch "Sketch27" plane through (0, 23.9, -20.1347) normal (0, 1, 0) x (1, 0, 0)
  line L0 (7.7562, 9.1565) -> (8.8598, 10.315)
  line L1 (8.8598, 10.315) -> (9.8734, 9.3493)
  line L2 (9.8734, 9.3493) -> (8.7698, 8.1908)
  circle A0 centre (0, 0) radius 12
  line L3 (7.7562, 9.1565) -> (8.7698, 8.1908) construction
  line L4 (8.263, 8.6737) -> (9.5575, 10.0325) construction
  line L5 (7.5596, 9.372) -> (7.5854, 9.3474) construction
  line L6 (7.5854, 9.3474) -> (8.9291, 8.0673) construction
  line L7 (0, 0) -> (0, 17.2564) construction
  line L8 (-7.7562, 9.1565) -> (-8.8598, 10.315)
  line L9 (-8.8598, 10.315) -> (-9.8734, 9.3493)
  line L10 (-7.7562, 9.1565) -> (-8.7698, 8.1908) construction
  line L11 (-9.8734, 9.3493) -> (-8.7698, 8.1908)
  line L12 (-8.263, 8.6737) -> (-9.5575, 10.0325) construction
  line L13 (-10.2373, -6.2608) -> (-11.0585, -6.8314)
  line L14 (-11.0585, -6.8314) -> (-10.2596, -7.9812)
  line L15 (-10.2596, -7.9812) -> (-9.4384, -7.4105)
  line L16 (-10.2373, -6.2608) -> (-9.4384, -7.4105) construction
  line L17 (-9.8379, -6.8357) -> (-14.5793, -10.1302) construction
  line L18 (-11.9013, -3.9018) -> (-8.4134, -8.9216) construction
  spline S0 degree 2 poles (-11.0585, -6.8314) (-16.1915, -6.3815) (-16.1298, -10.8902) knots 0 0 0 0.701787 0.701787 0.701787 weights 1 0.594412 1
  line L19 (-16.1298, -10.8902) -> (-15.3309, -12.0399)
  spline S1 degree 2 poles (-10.2596, -7.9812) (-14.0915, -8.4814) (-15.3309, -12.0399) knots 0 0 0 0.704179 0.704179 0.704179 weights 1 2.110661 1
  line L20 (16.1298, -10.8902) -> (15.3309, -12.0399)
  line L21 (10.2373, -6.2608) -> (9.4384, -7.4105) construction
  line L22 (11.9013, -3.9018) -> (8.4134, -8.9216) construction
  line L23 (9.8379, -6.8357) -> (14.5793, -10.1302) construction
  line L24 (11.0585, -6.8314) -> (10.2596, -7.9812)
  line L25 (10.2596, -7.9812) -> (9.4384, -7.4105)
  line L26 (10.2373, -6.2608) -> (11.0585, -6.8314)
  spline S2 degree 2 poles (11.0585, -6.8314) (16.1915, -6.3815) (16.1298, -10.8902) knots 0 0 0 0.701787 0.701787 0.701787 weights 1 0.594412 1
  spline S3 degree 2 poles (10.2596, -7.9812) (14.0915, -8.4814) (15.3309, -12.0399) knots 0 0 0 0.704179 0.704179 0.704179 weights 1 2.110661 1
  dimension "d216" = 1.6
  dimension "d217" = 1.4
  dimension "d226" = 1
  constraint perpendicular L0 L1
  constraint perpendicular L1 L2
  constraint coincident L0.start A0
  constraint coincident L2.end A0
  constraint midpoint L3 L4.start
  constraint perpendicular L3 L4
  constraint parallel L3 L5
  constraint perpendicular L4 L6
  constraint tangent A0 L6
  constraint parallel L1 L6
  constraint coincident A0.centre L7.start
  constraint vertical L7
  constraint symmetric L0.start L7 L8.start
  constraint symmetric L0.end L7 L8.end
  constraint symmetric L1.end L7 L9.end
  constraint symmetric L2.end L7 L10.end
  constraint symmetric L4.start L7 L12.start
  constraint symmetric L4.end L7 L12.end
  constraint coincident A0 L13.start
  constraint coincident A0 L15.end
  constraint parallel L13 L15
  constraint parallel L14 L16
  constraint midpoint L16 L17.start
  constraint perpendicular L16 L17
  constraint perpendicular L17 L18
  constraint tangent A0 L18
  constraint perpendicular L13 L14
  constraint equal L1 L14
  constraint parallel L14 L19
  constraint equal L14 L19
  constraint symmetric L7 L13.start L21.start
  constraint symmetric L7 L13.end L24.start
  constraint symmetric L7 L14.end L24.end
  constraint symmetric L7 L15.end L21.end
  constraint symmetric L7 L17.start L23.start
  constraint symmetric L7 L17.end L23.end
  constraint symmetric L7 L18.start L22.start
  constraint symmetric L7 L18.end L22.end
  constraint symmetric L7 S0.end L20.start
  constraint symmetric L7 S0 S2
  constraint symmetric L7 L19.end L20.end
  constraint symmetric L7 S1 S3
  measures "d216" distance of L1.end L2.end
  measures "d217" distance of L0.end L1.end
  measures "d226" distance of L13.start L13.end
extrude "Extrude8'" add sketch "Sketch27" against normal up to surface (21.4 mm away) separate body contours L0 L1 L2 A0 | A0 L8 L9 L11 | A0 L24 L25 L26 | A0 L13 L14 L15 | L20 L24 S2 S3 | L14 S0 L19 S1 makes body 10 at (8.1241, 9.6333, -29.6774) makes body 11 at (-8.1241, 9.6333, -29.6774) makes body 12 at (-13.4001, 13.2, -12.8982) makes body 13 at (13.4001, 13.2, -12.8982)
copy_body "CutPasteBodies2" bodies 11 10 removing the originals makes body 14 makes body 15 in component "Exchanger"
copy_body "CutPasteBodies3" bodies 12 13 removing the originals makes body 16 makes body 17 in component "Exchanger"
ref_plane "WorkPlane27" through (0, 24, -20.9985) normal (0, -1, 0) x (-1, 0, 0)
sketch "Sketch28" plane through (0, 24, -19.1261) normal (0, -1, 0) x (1, 0, 0)
  circle A0 centre (0, -1.0086) radius 10.1
  circle A1 centre (0, -1.0086) radius 10.5
  circle A2 centre (0, -1.0086) radius 8.6
  point P0 (0, -1.0086)
  dimension "d222" = 0.4
  dimension "d223" = 1.5
  constraint coincident P0 A0.centre
  constraint concentric A0 A2
  measures "d222" distance of A0 A1
  measures "d223" distance of A0 A2
extrude "Extrude2'''" add sketch "Sketch28" along normal blind 2 contours A0 bodies 7 in component "Roof"
fillet "Fillet6'" radius 1 2 edges at (-9.8734, 13.2, -29.4841) (9.8734, 13.2, -29.4841) on bodies 14 15 in component "Exchanger"
fillet "Fillet7" radius 2.5 4 edges at (-11.0585, 13.2, -13.3033) (-10.2596, 13.2, -12.1536) (11.0585, 13.2, -13.3033) (10.2596, 13.2, -12.1536) on bodies 16 17 in component "Exchanger"
fillet "Fillet8'" radius 2 2 edges at (-16.1298, 13.2, -9.2445) (16.1298, 13.2, -9.2445) on bodies 16 17 in component "Exchanger"
fillet "Fillet9'" radius 3 5 edges at (-6.5, 7.7228, -29.3014) (6.5, 7.7228, -29.3014) (-6.5, 18.6772, -29.3014) (6.5, 18.6772, -29.3014) (6.5, 7.7228, -29.3014) on bodies 4 in component "Exchanger"
ref_plane "WorkPlane28" through (0, -2, -33.4689) normal (0, -1, 0) x (1, 0, 0)
sketch "Sketch29" plane through (0, -2, -33.4689) normal (0, -1, 0) x (1, 0, 0)
  line L0 (-6.25, -3.3181) -> (6.25, -3.3181)
  line L1 (-6.25, -4.0398) -> (-6.25, 4.5803)
  line L2 (6.25, 4.5803) -> (6.25, -4.0398)
  line L3 (-6.8698, -3.3181) -> (0, -11.3181)
  line L4 (0, -11.3181) -> (6.8698, -3.3181)
  line L5 (6.8698, -3.3181) -> (-6.8698, -3.3181)
  line L6 (-26.6187, 19.6799) -> (0, -11.3181)
  line L7 (26.6187, 19.6799) -> (0, -11.3181)
  point P0 (0, -11.3181)
  dimension "d255" = 8
  constraint horizontal L0
  constraint coincident L0.end L2
  constraint horizontal L5
  constraint coincident L3.start L6
  constraint coincident P0 L3.end
  constraint coincident L4.end L7
  constraint coincident L0 L4.end
  measures "d255" distance of P0 L5
extrude "Extrude6'''" add sketch "Sketch29" along normal blind 4 bodies 8 in component "Motor Casing"
ref_plane "WorkPlane29" through (0, -2, -32.0022) normal (0, -1, 0) x (1, 0, 0)
sketch "Sketch30" plane through (0, -2, -32.0022) normal (0, -1, 0) x (1, 0, 0)
  line L0 (-6.25, 26.7522) -> (6.25, 26.7522)
  line L1 (6.25, 26.7522) -> (6.25, 20.3674)
  line L2 (6.25, 20.3674) -> (-6.25, 20.3674)
  line L3 (-6.25, 20.3674) -> (-6.25, 26.7522)
  arc A0 (6.25, 17.6283) -> (-6.25, 17.6283) centre (0, 11.8674) ccw
  line L4 (-6.25, 23.7522) -> (-6.25, 29.7522)
  line L5 (-6.25, 26.7522) -> (6.25, 26.7522)
  line L6 (6.25, 29.7522) -> (6.25, 23.7522)
  constraint horizontal L0
  constraint vertical L1
  constraint horizontal L2
  constraint vertical L3
  constraint tangent L2 A0
  constraint coincident L0.start L4
  constraint coincident L0.start L5
  constraint coincident L0.end L6
extrude "Extrude7''" add sketch "Sketch30" along normal up to surface (4 mm away) bodies 8 in component "Motor Casing"
fillet "Fillet10'" radius 1.5 4 edges at (-3.7, 5, -24.6347) (-3.7, 5, -15.6347) (3.7, 5, -24.6347) (3.7, 5, -15.6347) on bodies 6 in component "Exchanger"
fillet "Fillet21" radius 0.5 2 edges at (-12.3, 13, -20.1233) (12.3, 13, -20.1233) on bodies 2 in component "Casing"
fillet "Fillet22" radius 0.5 2 edges at (1.9495, 13, -32.2753) (-1.9495, 13, -32.2753) on bodies 2 in component "Casing"
fillet "Fillet23" radius 7 3 edges at (0, 12, -44.787) (26.6187, 12, -13.789) (-26.6187, 12, -13.789) on bodies 2 in component "Casing"
fillet "Fillet7'" radius 7 2 edges at (26.6187, -1, -13.789) (-26.6187, -1, -13.789) on bodies 8 in component "Motor Casing"
ref_plane "WorkPlane30" through (-3.125, -2, -13.0043) normal (0, -1, 0) x (1, 0, 0)
sketch "Sketch31" plane through (-3.125, -2, -13.0043) normal (0, -1, 0) x (1, 0, 0)
  line L0 (-3.125, 1.3696) -> (9.375, 1.3696)
  line L1 (9.375, 1.3696) -> (9.375, -1.6304)
  line L2 (9.375, -1.6304) -> (-3.125, -1.6304)
  line L3 (-3.125, -1.6304) -> (-3.125, 1.3696)
  line L4 (9.375, 1.3696) -> (-3.125, 1.3696)
  line L5 (-3.125, 0.7543) -> (-3.125, 4.7543)
  dimension "d265" = 3
  constraint horizontal L0
  constraint vertical L1
  constraint horizontal L2
  constraint vertical L3
  constraint coincident L0.start L4
  constraint coincident L0.start L5
  constraint coincident L0.end L1.start
  measures "d265" distance of L0.start L2.end
extrude "Extrude8''" add sketch "Sketch31" along normal up to surface (4 mm away) and the other way up to surface (2 mm away) bodies 8 in component "Motor Casing"
ref_plane "WorkPlane31" through (0, -6, -40.787) normal (0, -1, 0) x (0, 0, -1)
sketch "Sketch32" plane through (0, -6, -40.787) normal (0, -1, 0) x (1, 0, 0)
  line L0 (-6.25, 4) -> (6.25, 4)
  line L1 (6.25, 4) -> (6.25, -4)
  line L2 (6.25, -4) -> (-6.25, -4)
  line L3 (-6.25, -4) -> (-6.25, 4)
  line L4 (6.25, 11.8984) -> (6.25, 3.2782)
  line L5 (6.25, 4) -> (-6.25, 4)
  line L6 (-6.25, 3.2782) -> (-6.25, 11.8984)
  point P0 (0, -4)
  constraint horizontal L0
  constraint vertical L1
  constraint horizontal L2
  constraint vertical L3
  constraint coincident L2 P0
  constraint coincident L0.end L4
  constraint coincident L0.end L5
  constraint coincident L0.start L6
extrude "Extrude9" add sketch "Sketch32" against normal up to surface (6 mm away) bodies 8 in component "Motor Casing"
fillet "Fillet9''" radius 3 2 edges at (-6.25, -3, -44.787) (6.25, -3, -44.787) on bodies 8 in component "Motor Casing"
component "Exchanger" placed x (0.866025, 0, -0.5) y (0, 1, 0) z (0.5, 0, 0.866025) at (10.0674, 0, -2.6975)
component "Casing" placed x (1, 0, 0) y (0, 1, 0) z (0, 0, 1) at (0, 0, 0)
component "Roof" placed x (1, 0, 0) y (0, 1, 0) z (0, 0, 1) at (0, 0, 0)
component "Motor Casing" placed x (1, 0, 0) y (0, 1, 0) z (0, 0, 1) at (0, 0, 0)
component "Adapter 15-15" placed x (1, 0, 0) y (0, 1, 0) z (0, 0, 1) at (0, 0, 0)
